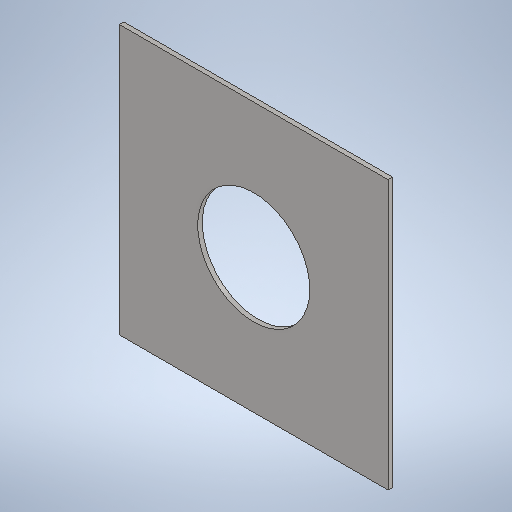
# Autodesk Inventor part: Крепление корпуса 2.0
Saved by Autodesk Inventor 2025 (Build 290162010, 162A)
## iProperties
Created: 2024-04-10
Part Number: Крепление корпуса 2.0
Material: Stainless Steel
Document SubType Name: Sheet Metal
Designer: admin
Density: 8 g/cm^3
Sheet Metal Rule: AISI304 2mm Die16
Appearance: Semi-Polished
Stock Number: Крепление корпуса 2.0
Author: admin
Autodesk Inventor part; units mm, degrees
ref_plane "YZ Plane" through (0, 0, 0) normal (1, 0, 0) x (0, 1, 0)
ref_plane "XZ Plane" through (0, 0, 0) normal (0, 1, 0) x (-1, 0, 0)
ref_plane "XY Plane" through (0, 0, 0) normal (0, 0, 1) x (1, 0, 0)
sketch "Sketch1" plane through (0, 0, 0) normal (0, 0, 1) x (1, 0, 0)
  line L0 (-60, 60) -> (-60, -60)
  line L1 (-60, -60) -> (60, -60)
  line L2 (60, -60) -> (60, 60)
  circle A0 centre (0, 0) radius 25
  line L3 (-60, 60) -> (60, 60)
  point P0 (0, -60)
  dimension "d4" = 120
  dimension "d13" = 50
  dimension "d14" = 120
  dimension "d15" = 60
  constraints: 8 end point, 2 perpendicular, 1 centre point, 1 coincident, 1 horizontal, 1 midpoint, 1 parallel, 1 vertical, 1 vertical alignment
  measures "d4" distance of L0.end L1.end
  measures "d13" diameter of A0
  measures "d14" distance of L1.end L2.end
  measures "d15" distance of point (0, -60) point (0, 0)
extrude "Extrusion1" add sketch "Sketch1" along normal blind 2
equation "\"d4\" = Ширина_крепления_корпуса"
equation "\"d14\" = Длина_крепления_корпуса"
equation "\"d15\" = 0.5 * Длина_крепления_корпуса"
equation "\"d5\" = Thickness"
equation "\"BendReliefWidth\" = Thickness"
equation "\"BendReliefDepth\" = 0.5 * Thickness"
equation "\"CornerReliefSize\" = 4 * Thickness"
equation "\"MinimumRemnant\" = 2 * Thickness"
equation "\"TransitionRadius\" = BendRadius"
equation "\"JacobiRadiusSize\" = BendRadius"
equation "\"GapSize\" = Thickness"
equation "\"Ширина_крепления_корпуса\" = 120"
equation "\"Длина_крепления_корпуса\" = 120"
equation "\"Thickness\" = 2"
equation "\"BendRadius\" = 2.75"
body "Solid1"
